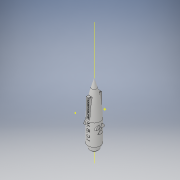
# Autodesk Inventor part: Pencil tooper
Saved by Autodesk Inventor 2018 (Build 220112000, 112)
## iProperties
Created: 2019-05-21
Part Number: Pencil tooper
Material: Generic
Document SubType Name: Modeling
Designer: 10043883
Density: 1 g/cm^3
Appearance: Default
Author: 10043883
Autodesk Inventor part; units mm, degrees
ref_plane "YZ Plane" through (0, 0, 0) normal (1, 0, 0) x (0, 1, 0)
sketch "Sketch1" plane through (0, 0, 0) normal (0, 0, 1) x (1, 0, 0)
  line L0 (0, 36.6275) -> (57.853, 36.6275) construction
  line L1 (25.9989, -2.9024) -> (51.3989, -2.9024)
  line L2 (25.9989, -2.9024) -> (51.3989, -2.9024)
  line L3 (51.3989, -2.9024) -> (51.3989, 38.3311)
  line L4 (51.3989, 38.3311) -> (25.9989, 38.3311)
  line L5 (25.9989, 38.3311) -> (25.9989, -2.9024)
  line L6 (38.6989, -2.9024) -> (38.6989, 38.3311)
  line L7 (25.9989, 38.3311) -> (38.6989, 82.474)
  line L8 (38.6989, 82.474) -> (51.3989, 38.3311)
  line L9 (38.6989, 82.474) -> (38.6989, 38.3311)
  line L10 (51.3989, -2.9024) -> (25.9989, -2.9024)
  line L11 (25.9989, -2.9024) -> (25.9989, -44.3081)
  line L12 (25.9989, -44.3081) -> (51.3989, -44.3081)
  line L13 (51.3989, -44.3081) -> (51.3989, -2.9024)
  line L14 (38.6989, -2.9024) -> (38.6989, -44.3081)
  point P0 (0, 0)
  point P1 (60.1022, 36.6275)
  point P2 (86.4535, -44.3081)
  dimension "d42" = 25.4
  constraints: 30 end point, 4 horizontal, 4 midpoint, 4 parallel, 3 point on line, 2 perpendicular, 1 collinear
  measures "d42" distance of L11.end L12.end
sketch "Sketch2" plane through (0, 0, 0) normal (0, 0, 1) x (1, 0, 0)
  point P0 (0, 0)
revolve "Revolution2" add sketch "Sketch1" angle 360 about axis through (38.6989, -2.9024, 0) along (0, 1, 0) contours L5 L4 L6 L1
revolve "Revolution5" add sketch "Sketch1" angle 360 about axis through (38.6989, 82.474, 0) along (0, -1, 0) contours L1 L14 L12 L11 | L7 L9 L4
hole "Hole4" at (38.6989, -44.3081, 0) direction (0, 1, 0) diameter 10.16 depth 38.1 tip angle 60
ref_plane "Work Plane9" through (38.6989, 17.7144, 12.7) normal (0, 0, -1) x (-1, 0, 0)
ref_plane "Work Plane8" through (38.6989, -44.3081, 0) normal (0, 0, -1) x (0, 1, 0)
sketch "Sketch6" plane through (38.6989, 17.7144, 12.7) normal (0, 0, -1) x (-1, 0, 0)
  line L0 (-3.4954, -41.6942) -> (-3.4954, -36.5195) construction
  line L1 (-3.4954, -36.5195) -> (31.8486, -36.5195) construction
  line L2 (31.8486, -36.5195) -> (31.8486, -41.6942) construction
  line L3 (31.8486, -41.6942) -> (-3.4954, -41.6942) construction
  line L4 (2.6638, -40.6345) -> (-3.4322, -40.6345)
  line L5 (-3.4322, -40.6345) -> (-3.4322, -40.3039)
  line L6 (-3.4322, -40.3039) -> (2.6638, -40.3039)
  line L7 (2.6638, -40.3039) -> (2.6638, -40.6345)
  line L8 (2.7805, -37.7275) -> (2.2846, -38.2525)
  line L9 (2.2846, -38.2525) -> (1.7791, -37.7275)
  line L10 (1.7791, -37.7275) -> (2.2846, -37.2073)
  line L11 (2.2846, -37.2073) -> (2.7805, -37.7275)
  line L12 (1.152, -30.7467) -> (1.8228, -31.087)
  line L13 (1.8228, -31.087) -> (2.4208, -31.7044)
  line L14 (2.4208, -31.7044) -> (2.7173, -32.3461)
  line L15 (2.7173, -32.3461) -> (2.7173, -33.5857)
  line L16 (2.7173, -33.5857) -> (2.4208, -34.2225)
  line L17 (2.4208, -34.2225) -> (1.8228, -34.8447)
  line L18 (1.8228, -34.8447) -> (1.22, -35.1413)
  line L19 (1.22, -35.1413) -> (0.345, -35.4475)
  line L20 (0.345, -35.4475) -> (-1.1085, -35.4475)
  line L21 (-1.1085, -35.4475) -> (-1.9884, -35.1413)
  line L22 (-1.9884, -35.1413) -> (-2.5912, -34.8447)
  line L23 (-2.5912, -34.8447) -> (-3.1891, -34.2225)
  line L24 (-3.1891, -34.2225) -> (-3.4954, -33.5857)
  line L25 (-3.4954, -33.5857) -> (-3.4954, -32.3461)
  line L26 (-3.4954, -32.3461) -> (-3.1891, -31.7044)
  line L27 (-3.1891, -31.7044) -> (-2.5912, -31.087)
  line L28 (-2.5912, -31.087) -> (-1.9203, -30.7467)
  line L29 (-1.9203, -30.7467) -> (-1.7599, -31.0384)
  line L30 (-1.7599, -31.0384) -> (-2.3919, -31.369)
  line L31 (-2.3919, -31.369) -> (-2.9169, -31.9086)
  line L32 (-2.9169, -31.9086) -> (-3.1697, -32.4238)
  line L33 (-3.1697, -32.4238) -> (-3.1697, -33.503)
  line L34 (-3.1697, -33.503) -> (-2.9169, -34.0232)
  line L35 (-2.9169, -34.0232) -> (-2.3919, -34.5628)
  line L36 (-2.3919, -34.5628) -> (-1.8669, -34.8399)
  line L37 (-1.8669, -34.8399) -> (-1.0647, -35.1121)
  line L38 (-1.0647, -35.1121) -> (0.2964, -35.1121)
  line L39 (0.2964, -35.1121) -> (1.0985, -34.8399)
  line L40 (1.0985, -34.8399) -> (1.6235, -34.5628)
  line L41 (1.6235, -34.5628) -> (2.1485, -34.0232)
  line L42 (2.1485, -34.0232) -> (2.4013, -33.503)
  line L43 (2.4013, -33.503) -> (2.4013, -32.4238)
  line L44 (2.4013, -32.4238) -> (2.1485, -31.9086)
  line L45 (2.1485, -31.9086) -> (1.6235, -31.369)
  line L46 (1.6235, -31.369) -> (0.9916, -31.0384)
  line L47 (0.9916, -31.0384) -> (1.152, -30.7467)
  line L48 (2.7805, -27.3244) -> (2.2846, -27.8494)
  line L49 (2.2846, -27.8494) -> (1.7791, -27.3244)
  line L50 (1.7791, -27.3244) -> (2.2846, -26.8042)
  line L51 (2.2846, -26.8042) -> (2.7805, -27.3244)
  line L52 (-0.5251, -21.4569) -> (-0.389, -21.0291)
  line L53 (-0.389, -21.0291) -> (-0.0585, -20.6839)
  line L54 (-0.0585, -20.6839) -> (0.5638, -20.368)
  line L55 (0.5638, -20.368) -> (1.4825, -20.368)
  line L56 (1.4825, -20.368) -> (2.0999, -20.6839)
  line L57 (2.0999, -20.6839) -> (2.4256, -21.0291)
  line L58 (2.4256, -21.0291) -> (2.7173, -21.9576)
  line L59 (2.7173, -21.9576) -> (2.7173, -24.7528)
  line L60 (2.7173, -24.7528) -> (-3.4954, -24.7528)
  line L61 (-3.4954, -24.7528) -> (-3.4954, -21.9576)
  line L62 (-3.4954, -21.9576) -> (-3.194, -21.0291)
  line L63 (-3.194, -21.0291) -> (-2.8731, -20.6839)
  line L64 (-2.8731, -20.6839) -> (-2.246, -20.368)
  line L65 (-2.246, -20.368) -> (-1.6092, -20.368)
  line L66 (-1.6092, -20.368) -> (-0.987, -20.6839)
  line L67 (-0.987, -20.6839) -> (-0.6613, -21.0291)
  line L68 (-0.6613, -21.0291) -> (-0.5251, -21.4569)
  line L69 (-0.3599, -22.0062) -> (-0.3599, -24.4222)
  line L70 (-0.3599, -24.4222) -> (2.4013, -24.4222)
  line L71 (2.4013, -24.4222) -> (2.4013, -22.0062)
  line L72 (2.4013, -22.0062) -> (2.1437, -21.2041)
  line L73 (2.1437, -21.2041) -> (1.9055, -20.9659)
  line L74 (1.9055, -20.9659) -> (1.3999, -20.7034)
  line L75 (1.3999, -20.7034) -> (0.6367, -20.7034)
  line L76 (0.6367, -20.7034) -> (0.136, -20.9659)
  line L77 (0.136, -20.9659) -> (-0.1022, -21.2041)
  line L78 (-0.1022, -21.2041) -> (-0.3599, -22.0062)
  line L79 (-0.6856, -24.4222) -> (-0.6856, -22.0062)
  line L80 (-0.6856, -22.0062) -> (-0.9432, -21.2041)
  line L81 (-0.9432, -21.2041) -> (-1.1863, -20.9659)
  line L82 (-1.1863, -20.9659) -> (-1.687, -20.7034)
  line L83 (-1.687, -20.7034) -> (-2.1683, -20.7034)
  line L84 (-2.1683, -20.7034) -> (-2.6738, -20.9659)
  line L85 (-2.6738, -20.9659) -> (-2.912, -21.2041)
  line L86 (-2.912, -21.2041) -> (-3.1697, -22.0062)
  line L87 (-3.1697, -22.0062) -> (-3.1697, -24.4222)
  line L88 (-3.1697, -24.4222) -> (-0.6856, -24.4222)
  line L89 (2.7805, -16.9213) -> (2.2846, -17.4463)
  line L90 (2.2846, -17.4463) -> (1.7791, -16.9213)
  line L91 (1.7791, -16.9213) -> (2.2846, -16.4012)
  line L92 (2.2846, -16.4012) -> (2.7805, -16.9213)
  line L93 (2.6638, -9.3864) -> (2.6638, -9.717)
  line L94 (2.6638, -9.717) -> (-2.4551, -9.717)
  line L95 (-2.4551, -9.717) -> (2.6638, -11.7295)
  line L96 (2.6638, -11.7295) -> (2.6638, -12.0018)
  line L97 (2.6638, -12.0018) -> (-2.4551, -14.0192)
  line L98 (-2.4551, -14.0192) -> (2.6638, -14.0192)
  line L99 (2.6638, -14.0192) -> (2.6638, -14.3497)
  line L100 (2.6638, -14.3497) -> (-3.4322, -14.3497)
  line L101 (-3.4322, -14.3497) -> (-3.4322, -14.0483)
  line L102 (-3.4322, -14.0483) -> (2.1145, -11.8656)
  line L103 (2.1145, -11.8656) -> (-3.4322, -9.6878)
  line L104 (-3.4322, -9.6878) -> (-3.4322, -9.3864)
  line L105 (-3.4322, -9.3864) -> (2.6638, -9.3864)
  point P0 (38.6989, -17.7144)
  constraints: 2 other
extrude "Extrusion3" add sketch "Sketch6" along normal blind 25.4
ref_plane "Work Plane10" through (51.3989, -2.9024, 0) normal (1, 0, 0) x (0, 1, 0)
fillet "Fillet5" radius 196.85 1 edges at (51.3989, 38.3311, 0)
sketch "Sketch7" plane through (51.3989, -2.9024, 0) normal (1, 0, 0) x (0, 1, 0)
  line L0 (0.2488, 2.5647) -> (0.2488, -2.5647) projected
  circle A0 centre (0.2488, 0) radius 10.3788
  arc A1 (8.5027, 1.9887) -> (1.1594, 9.0888) centre (-0.0471, 0.4934) ccw
  line L1 (1.1594, 9.0888) -> (0.276, 3.4875)
  line L2 (8.5027, 1.9887) -> (2.844, 1.4137)
  arc A2 (2.844, 1.4137) -> (0.276, 3.4875) centre (-0.4963, -0.0957) ccw
  circle A3 centre (0.2488, 0) radius 2.2322
  arc A4 (0.8722, -9.1023) -> (8.4313, -2.2325) centre (-0.0683, -0.4738) ccw
  line L3 (8.4313, -2.2325) -> (2.8987, -0.9894)
  line L4 (0.8722, -9.1023) -> (0.6635, -3.4182)
  arc A5 (0.6635, -3.4182) -> (2.8987, -0.9894) centre (-0.6272, 0.0125) ccw
  arc A6 (-7.9804, 4.8535) -> (-7.5597, -4.9877) centre (-0.6296, 0.2381) ccw
  line L5 (-7.5597, -4.9877) -> (-2.9749, -1.6509)
  line L6 (-7.9804, 4.8535) -> (-2.9749, 1.4137)
  arc A7 (-2.9749, 1.4137) -> (-2.9749, -1.6509) centre (0.355, -0.1186) ccw
  point P0 (2.9024, 0)
  constraints: 12 end point, 12 point on circle, 8 centre point, 1 coincident, 1 midpoint
extrude "Extrusion4" add sketch "Sketch7" against normal blind 25.4 contours A3 L0 | L0 A3 | L2 A2 L1 A1 | L4 A5 L3 A4 | L6 A7 L5 A6
chamfer "Chamfer1" distance 5.715 angle 45 1 edges at (51.3989, -44.3081, 0)
chamfer "Chamfer2" distance 5.715 angle 45 1 edges at (51.3989, -38.5931, 0)
sketch "Sketch8" plane through (38.6989, 17.7144, 12.7) normal (0, 0, -1) x (-1, 0, 0)
  line L0 (-3.3915, 35.5657) -> (3.9696, 35.5657)
  line L1 (3.9696, 35.5657) -> (3.9696, -3.0269)
  line L2 (3.9696, -3.0269) -> (-3.3915, -3.0269)
  line L3 (-3.3915, -3.0269) -> (-3.3915, 35.5657)
  point P0 (38.6989, -17.7144)
  constraints: 8 end point, 2 parallel, 1 horizontal, 1 perpendicular
extrude "Extrusion5" add sketch "Sketch8" along normal blind 25.4
sketch "Sketch9" plane through (38.6989, 17.7144, 12.7) normal (0, 0, 1) x (1, 0, 0)
  line L0 (2.0658, 35.4953) -> (2.0658, 4.9175) construction
  line L1 (2.0658, 4.9175) -> (-2.3913, 4.9175) construction
  line L2 (-2.3913, 4.9175) -> (-2.3913, 35.4953) construction
  line L3 (-2.3913, 35.4953) -> (2.0658, 35.4953) construction
  line L4 (1.4194, 33.6183) -> (-0.8902, 33.6183)
  spline S0 degree 2 poles (-0.8902, 33.6183) (-0.9598, 33.6183) (-1.0319, 33.5562) (-1.0543, 33.4741) knots 0 0 0 1 2 2 2
  line L5 (-1.0543, 33.4741) -> (-1.1264, 33.4741)
  line L6 (-1.1264, 33.4741) -> (-1.1264, 34.4288)
  line L7 (-1.1264, 34.4288) -> (-1.0543, 34.4288)
  spline S1 degree 2 poles (-1.0543, 34.4288) (-1.0319, 34.3468) (-0.9598, 34.2846) (-0.8902, 34.2846) knots 0 0 0 1 2 2 2
  line L8 (-0.8902, 34.2846) -> (1.4194, 34.2846)
  line L9 (1.4194, 34.2846) -> (1.4194, 35.2293)
  spline S2 degree 2 poles (1.4194, 35.2293) (1.4194, 35.2965) (1.3573, 35.3686) (1.2752, 35.3909) knots 0 0 0 1 2 2 2
  line L10 (1.2752, 35.3909) -> (1.2752, 35.463)
  line L11 (1.2752, 35.463) -> (2.0658, 35.463)
  line L12 (2.0658, 35.463) -> (2.0658, 35.3909)
  spline S3 degree 2 poles (2.0658, 35.3909) (1.9838, 35.3661) (1.9216, 35.2965) (1.9216, 35.2293) knots 0 0 0 1 2 2 2
  line L13 (1.9216, 35.2293) -> (1.9216, 32.6761)
  spline S4 degree 2 poles (1.9216, 32.6761) (1.9216, 32.6065) (1.9838, 32.5344) (2.0658, 32.512) knots 0 0 0 1 2 2 2
  line L14 (2.0658, 32.512) -> (2.0658, 32.4399)
  line L15 (2.0658, 32.4399) -> (1.2752, 32.4399)
  line L16 (1.2752, 32.4399) -> (1.2752, 32.512)
  spline S5 degree 2 poles (1.2752, 32.512) (1.3573, 32.5344) (1.4194, 32.6065) (1.4194, 32.6736) knots 0 0 0 1 2 2 2
  line L17 (1.4194, 32.6736) -> (1.4194, 33.6183)
  line L18 (-0.4999, 30.2968) -> (-0.4999, 31.4429)
  line L19 (-0.4999, 31.4429) -> (-0.7733, 31.5722)
  spline S6 degree 2 poles (-0.7733, 31.5722) (-0.8728, 31.6195) (-0.9275, 31.6195) knots 0 0 0 1 1 1
  spline S7 degree 2 poles (-0.9275, 31.6195) (-1.0344, 31.6195) (-1.0642, 31.4753) knots 0 0 0 1 1 1
  line L20 (-1.0642, 31.4753) -> (-1.1264, 31.4753)
  line L21 (-1.1264, 31.4753) -> (-1.1264, 32.3976)
  line L22 (-1.1264, 32.3976) -> (-1.0642, 32.3976)
  spline S8 degree 2 poles (-1.0642, 32.3976) (-1.0518, 32.3131) (-0.9747, 32.2311) (-0.8628, 32.1739) knots 0 0 0 1 2 2 2
  line L23 (-0.8628, 32.1739) -> (0.9869, 31.2615)
  spline S9 degree 2 poles (0.9869, 31.2615) (1.0913, 31.2093) (1.1708, 31.2093) knots 0 0 0 1 1 1
  spline S10 degree 2 poles (1.1708, 31.2093) (1.2603, 31.2093) (1.3125, 31.3336) knots 0 0 0 1 1 1
  line L24 (1.3125, 31.3336) -> (1.3747, 31.3336)
  line L25 (1.3747, 31.3336) -> (1.3747, 30.364)
  line L26 (1.3747, 30.364) -> (1.3125, 30.364)
  spline S11 degree 2 poles (1.3125, 30.364) (1.2628, 30.4858) (1.1609, 30.4858) knots 0 0 0 1 1 1
  spline S12 degree 2 poles (1.1609, 30.4858) (1.0863, 30.4858) (0.9794, 30.4311) knots 0 0 0 1 1 1
  line L27 (0.9794, 30.4311) -> (-0.8131, 29.4839)
  spline S13 degree 2 poles (-0.8131, 29.4839) (-0.9598, 29.4068) (-1.0468, 29.3173) (-1.0642, 29.2253) knots 0 0 0 1 2 2 2
  line L28 (-1.0642, 29.2253) -> (-1.1264, 29.2253)
  line L29 (-1.1264, 29.2253) -> (-1.1264, 30.2471)
  line L30 (-1.1264, 30.2471) -> (-1.0642, 30.2471)
  spline S14 degree 2 poles (-1.0642, 30.2471) (-1.0393, 30.1029) (-0.9275, 30.1029) knots 0 0 0 1 1 1
  spline S15 degree 2 poles (-0.9275, 30.1029) (-0.8579, 30.1029) (-0.7559, 30.1576) knots 0 0 0 1 1 1
  line L31 (-0.7559, 30.1576) -> (-0.4999, 30.2968)
  line L32 (-0.1493, 30.4758) -> (0.6512, 30.8836)
  line L33 (0.6512, 30.8836) -> (-0.1493, 31.2714)
  line L34 (-0.1493, 31.2714) -> (-0.1493, 30.4758)
  line L35 (-0.0971, 28.2731) -> (-0.8976, 28.2731)
  spline S16 degree 2 poles (-0.8976, 28.2731) (-0.9648, 28.2731) (-1.0393, 28.211) (-1.0642, 28.1289) knots 0 0 0 1 2 2 2
  line L36 (-1.0642, 28.1289) -> (-1.1264, 28.1289)
  line L37 (-1.1264, 28.1289) -> (-1.1264, 29.0165)
  line L38 (-1.1264, 29.0165) -> (-1.0642, 29.0165)
  spline S17 degree 2 poles (-1.0642, 29.0165) (-1.0443, 28.9369) (-0.9672, 28.8723) (-0.9001, 28.8723) knots 0 0 0 1 2 2 2
  line L39 (-0.9001, 28.8723) -> (1.1485, 28.8723)
  spline S18 degree 2 poles (1.1485, 28.8723) (1.2156, 28.8723) (1.2877, 28.9344) (1.3125, 29.0165) knots 0 0 0 1 2 2 2
  line L40 (1.3125, 29.0165) -> (1.3747, 29.0165)
  line L41 (1.3747, 29.0165) -> (1.3747, 27.3781)
  spline S19 degree 2 poles (1.3747, 27.3781) (1.3747, 27.0574) (1.3101, 26.7243) (1.2255, 26.5925) knots 0 0 0 1 2 2 2
  spline S20 degree 2 poles (1.2255, 26.5925) (1.049, 26.3215) (0.6512, 26.3215) knots 0 0 0 1 1 1
  spline S21 degree 2 poles (0.6512, 26.3215) (0.3479, 26.3215) (0.0048, 26.6547) (-0.0698, 27.0251) knots 0 0 0 1 2 2 2
  line L42 (-0.0698, 27.0251) -> (-0.7311, 26.5527)
  spline S22 degree 2 poles (-0.7311, 26.5527) (-0.915, 26.421) (-1.0468, 26.2668) (-1.0642, 26.1699) knots 0 0 0 1 2 2 2
  line L43 (-1.0642, 26.1699) -> (-1.1264, 26.1699)
  line L44 (-1.1264, 26.1699) -> (-1.1264, 27.219)
  line L45 (-1.1264, 27.219) -> (-1.0642, 27.219)
  spline S23 degree 2 poles (-1.0642, 27.219) (-1.0319, 27.1046) (-0.9648, 27.1046) knots 0 0 0 1 1 1
  spline S24 degree 2 poles (-0.9648, 27.1046) (-0.915, 27.1046) (-0.8131, 27.1767) knots 0 0 0 1 1 1
  line L46 (-0.8131, 27.1767) -> (-0.0971, 27.674)
  line L47 (-0.0971, 27.674) -> (-0.0971, 28.2731)
  line L48 (0.3554, 28.2731) -> (0.3554, 27.3731)
  spline S25 degree 2 poles (0.3554, 27.3731) (0.3554, 27.1668) (0.4001, 27.0698) knots 0 0 0 1 1 1
  spline S26 degree 2 poles (0.4001, 27.0698) (0.4598, 26.9306) (0.6388, 26.9306) knots 0 0 0 1 1 1
  spline S27 degree 2 poles (0.6388, 26.9306) (0.7979, 26.9306) (0.9222, 27.1245) (0.9222, 27.3731) knots 0 0 0 1 2 2 2
  line L49 (0.9222, 27.3731) -> (0.9222, 28.2731)
  line L50 (0.9222, 28.2731) -> (0.3554, 28.2731)
  line L51 (-0.1617, 23.6216) -> (-0.1617, 24.1909)
  spline S28 degree 2 poles (-0.1617, 24.1909) (-0.1617, 24.263) (-0.2239, 24.3376) (-0.3059, 24.36) knots 0 0 0 1 2 2 2
  line L52 (-0.3059, 24.36) -> (-0.3059, 24.4196)
  line L53 (-0.3059, 24.4196) -> (0.3604, 24.4196)
  line L54 (0.3604, 24.4196) -> (0.3604, 24.36)
  spline S29 degree 2 poles (0.3604, 24.36) (0.2808, 24.3376) (0.2162, 24.263) (0.2162, 24.1934) knots 0 0 0 1 2 2 2
  line L55 (0.2162, 24.1934) -> (0.2162, 23)
  line L56 (0.2162, 23) -> (0.1515, 23)
  spline S30 degree 2 poles (0.1515, 23) (0.1291, 23.0796) (0.0446, 23.1442) (-0.0349, 23.1442) knots 0 0 0 1 2 2 2
  line L57 (-0.0349, 23.1442) -> (-0.562, 23.1442)
  spline S31 degree 2 poles (-0.562, 23.1442) (-0.6291, 23.1442) (-0.7062, 23.0796) (-0.7286, 23) knots 0 0 0 1 2 2 2
  line L58 (-0.7286, 23) -> (-0.7808, 23)
  spline S32 degree 2 poles (-0.7808, 23) (-1.1811, 23.7235) (-1.1811, 24.442) knots 0 0 0 1 1 1
  spline S33 degree 2 poles (-1.1811, 24.442) (-1.1811, 25.0635) (-0.8877, 25.4464) knots 0 0 0 1 1 1
  spline S34 degree 2 poles (-0.8877, 25.4464) (-0.7286, 25.6552) (-0.4899, 25.782) knots 0 0 0 1 1 1
  spline S35 degree 2 poles (-0.4899, 25.782) (-0.209, 25.9312) (0.1117, 25.9312) knots 0 0 0 1 1 1
  spline S36 degree 2 poles (0.1117, 25.9312) (0.5543, 25.9312) (0.8974, 25.6602) knots 0 0 0 1 1 1
  spline S37 degree 2 poles (0.8974, 25.6602) (1.4294, 25.2351) (1.4294, 24.4072) knots 0 0 0 1 1 1
  spline S38 degree 2 poles (1.4294, 24.4072) (1.4294, 24.0417) (1.2678, 23.5768) knots 0 0 0 1 1 1
  spline S39 degree 2 poles (1.2678, 23.5768) (1.2056, 23.3904) (1.2056, 23.3605) knots 0 0 0 1 1 1
  spline S40 degree 2 poles (1.2056, 23.3605) (1.2056, 23.3232) (1.2429, 23.271) knots 0 0 0 1 1 1
  line L59 (1.2429, 23.271) -> (1.2131, 23.2163)
  line L60 (1.2131, 23.2163) -> (0.5841, 23.5122)
  line L61 (0.5841, 23.5122) -> (0.609, 23.5669)
  spline S41 degree 2 poles (0.609, 23.5669) (0.6189, 23.5669) (0.6239, 23.5669) knots 0 0 0 1 1 1
  spline S42 degree 2 poles (0.6239, 23.5669) (0.7059, 23.5669) (0.7929, 23.731) knots 0 0 0 1 1 1
  spline S43 degree 2 poles (0.7929, 23.731) (0.957, 24.0368) (0.957, 24.3873) knots 0 0 0 1 1 1
  spline S44 degree 2 poles (0.957, 24.3873) (0.957, 24.7901) (0.7358, 25.0511) knots 0 0 0 1 1 1
  spline S45 degree 2 poles (0.7358, 25.0511) (0.5021, 25.3221) (0.1093, 25.3221) knots 0 0 0 1 1 1
  spline S46 degree 2 poles (0.1093, 25.3221) (-0.2612, 25.3221) (-0.4824, 25.0735) knots 0 0 0 1 1 1
  spline S47 degree 2 poles (-0.4824, 25.0735) (-0.7087, 24.8199) (-0.7087, 24.36) knots 0 0 0 1 1 1
  spline S48 degree 2 poles (-0.7087, 24.36) (-0.7087, 23.9224) (-0.5446, 23.6216) knots 0 0 0 1 1 1
  line L62 (-0.5446, 23.6216) -> (-0.1617, 23.6216)
  line L63 (-0.0623, 21.839) -> (-0.6739, 21.839)
  line L64 (-0.6739, 21.839) -> (-0.6739, 20.2504)
  spline S49 degree 2 poles (-0.6739, 20.2504) (-0.6739, 20.1832) (-0.6117, 20.1087) (-0.5297, 20.0863) knots 0 0 0 1 2 2 2
  line L65 (-0.5297, 20.0863) -> (-0.5297, 20.0241)
  line L66 (-0.5297, 20.0241) -> (-1.2706, 20.0241)
  line L67 (-1.2706, 20.0241) -> (-1.2706, 20.0863)
  spline S50 degree 2 poles (-1.2706, 20.0863) (-1.191, 20.1062) (-1.1264, 20.1832) (-1.1264, 20.2529) knots 0 0 0 1 2 2 2
  line L68 (-1.1264, 20.2529) -> (-1.1264, 22.5824)
  line L69 (-1.1264, 22.5824) -> (-1.0642, 22.5824)
  spline S51 degree 2 poles (-1.0642, 22.5824) (-1.0443, 22.5028) (-0.9672, 22.4382) (-0.9001, 22.4382) knots 0 0 0 1 2 2 2
  line L70 (-0.9001, 22.4382) -> (1.1485, 22.4382)
  spline S52 degree 2 poles (1.1485, 22.4382) (1.2156, 22.4382) (1.2877, 22.5003) (1.3125, 22.5824) knots 0 0 0 1 2 2 2
  line L71 (1.3125, 22.5824) -> (1.3747, 22.5824)
  line L72 (1.3747, 22.5824) -> (1.3747, 20.32)
  spline S53 degree 2 poles (1.3747, 20.32) (1.3747, 20.2504) (1.4368, 20.1758) (1.5189, 20.1534) knots 0 0 0 1 2 2 2
  line L73 (1.5189, 20.1534) -> (1.5189, 20.0937)
  line L74 (1.5189, 20.0937) -> (0.778, 20.0937)
  line L75 (0.778, 20.0937) -> (0.778, 20.1534)
  spline S54 degree 2 poles (0.778, 20.1534) (0.8601, 20.1758) (0.9222, 20.2504) (0.9222, 20.32) knots 0 0 0 1 2 2 2
  line L76 (0.9222, 20.32) -> (0.9222, 21.839)
  line L77 (0.9222, 21.839) -> (0.3728, 21.839)
  line L78 (0.3728, 21.839) -> (0.3728, 20.8943)
  spline S55 degree 2 poles (0.3728, 20.8943) (0.3728, 20.8272) (0.4349, 20.7526) (0.517, 20.7277) knots 0 0 0 1 2 2 2
  line L79 (0.517, 20.7277) -> (0.517, 20.668)
  line L80 (0.517, 20.668) -> (-0.2065, 20.668)
  line L81 (-0.2065, 20.668) -> (-0.2065, 20.7277)
  spline S56 degree 2 poles (-0.2065, 20.7277) (-0.1269, 20.7501) (-0.0623, 20.8247) (-0.0623, 20.8943) knots 0 0 0 1 2 2 2
  line L82 (-0.0623, 20.8943) -> (-0.0623, 21.839)
  line L83 (0.9222, 18.2664) -> (-0.8976, 18.2664)
  spline S57 degree 2 poles (-0.8976, 18.2664) (-0.9648, 18.2664) (-1.0393, 18.2043) (-1.0642, 18.1222) knots 0 0 0 1 2 2 2
  line L84 (-1.0642, 18.1222) -> (-1.1264, 18.1222)
  line L85 (-1.1264, 18.1222) -> (-1.1264, 19.0098)
  line L86 (-1.1264, 19.0098) -> (-1.0642, 19.0098)
  spline S58 degree 2 poles (-1.0642, 19.0098) (-1.0443, 18.9302) (-0.9672, 18.8656) (-0.8976, 18.8656) knots 0 0 0 1 2 2 2
  line L87 (-0.8976, 18.8656) -> (0.9222, 18.8656)
  line L88 (0.9222, 18.8656) -> (0.9222, 19.604)
  spline S59 degree 2 poles (0.9222, 19.604) (0.9222, 19.6736) (0.8576, 19.7482) (0.778, 19.7705) knots 0 0 0 1 2 2 2
  line L89 (0.778, 19.7705) -> (0.778, 19.8302)
  line L90 (0.778, 19.8302) -> (1.5189, 19.8302)
  line L91 (1.5189, 19.8302) -> (1.5189, 19.7705)
  spline S60 degree 2 poles (1.5189, 19.7705) (1.4393, 19.7507) (1.3747, 19.6761) (1.3747, 19.604) knots 0 0 0 1 2 2 2
  line L92 (1.3747, 19.604) -> (1.3747, 17.5281)
  spline S61 degree 2 poles (1.3747, 17.5281) (1.3747, 17.4584) (1.4368, 17.3839) (1.5189, 17.3615) knots 0 0 0 1 2 2 2
  line L93 (1.5189, 17.3615) -> (1.5189, 17.3018)
  line L94 (1.5189, 17.3018) -> (0.778, 17.3018)
  line L95 (0.778, 17.3018) -> (0.778, 17.3615)
  spline S62 degree 2 poles (0.778, 17.3615) (0.8576, 17.3839) (0.9222, 17.4584) (0.9222, 17.5281) knots 0 0 0 1 2 2 2
  line L96 (0.9222, 17.5281) -> (0.9222, 18.2664)
  spline S63 degree 2 poles (1.4294, 16.5585) (1.4294, 16.4043) (1.2156, 16.193) (1.0614, 16.193) knots 0 0 0 1 2 2 2
  spline S64 degree 2 poles (1.0614, 16.193) (0.9098, 16.193) (0.696, 16.4093) (0.696, 16.5585) knots 0 0 0 1 2 2 2
  spline S65 degree 2 poles (0.696, 16.5585) (0.696, 16.7126) (0.9123, 16.9264) (1.0639, 16.9264) knots 0 0 0 1 2 2 2
  spline S66 degree 2 poles (1.0639, 16.9264) (1.2156, 16.9264) (1.4269, 16.7151) (1.4294, 16.5585) knots 0 0 0 1 2 2 2
  spline S67 degree 2 poles (-0.4476, 16.5585) (-0.4476, 16.4043) (-0.6615, 16.193) (-0.8156, 16.193) knots 0 0 0 1 2 2 2
  spline S68 degree 2 poles (-0.8156, 16.193) (-0.9672, 16.193) (-1.1811, 16.4093) (-1.1811, 16.5585) knots 0 0 0 1 2 2 2
  spline S69 degree 2 poles (-1.1811, 16.5585) (-1.1811, 16.7126) (-0.9648, 16.9264) (-0.8131, 16.9264) knots 0 0 0 1 2 2 2
  spline S70 degree 2 poles (-0.8131, 16.9264) (-0.6615, 16.9264) (-0.4501, 16.7151) (-0.4476, 16.5585) knots 0 0 0 1 2 2 2
  line L97 (-1.1264, 13.7069) -> (0.9794, 14.8331)
  line L98 (0.9794, 14.8331) -> (-0.8902, 14.8331)
  spline S71 degree 2 poles (-0.8902, 14.8331) (-0.9598, 14.8331) (-1.0319, 14.7709) (-1.0543, 14.6889) knots 0 0 0 1 2 2 2
  line L99 (-1.0543, 14.6889) -> (-1.1264, 14.6889)
  line L100 (-1.1264, 14.6889) -> (-1.1264, 15.5864)
  line L101 (-1.1264, 15.5864) -> (-1.0543, 15.5864)
  spline S72 degree 2 poles (-1.0543, 15.5864) (-1.0319, 15.5043) (-0.9598, 15.4422) (-0.8902, 15.4422) knots 0 0 0 1 2 2 2
  line L102 (-0.8902, 15.4422) -> (1.6879, 15.4422)
  spline S73 degree 2 poles (1.6879, 15.4422) (1.7551, 15.4422) (1.8272, 15.5043) (1.8495, 15.5864) knots 0 0 0 1 2 2 2
  line L103 (1.8495, 15.5864) -> (1.9216, 15.5864)
  line L104 (1.9216, 15.5864) -> (1.9216, 14.4104)
  line L105 (1.9216, 14.4104) -> (1.8495, 14.4104)
  spline S74 degree 2 poles (1.8495, 14.4104) (1.8222, 14.5149) (1.7277, 14.5149) knots 0 0 0 1 1 1
  spline S75 degree 2 poles (1.7277, 14.5149) (1.683, 14.5149) (1.6233, 14.485) knots 0 0 0 1 1 1
  line L106 (1.6233, 14.485) -> (0.0546, 13.6547)
  line L107 (0.0546, 13.6547) -> (1.5984, 12.8119)
  spline S76 degree 2 poles (1.5984, 12.8119) (1.7004, 12.7547) (1.7476, 12.7547) knots 0 0 0 1 1 1
  spline S77 degree 2 poles (1.7476, 12.7547) (1.8396, 12.7547) (1.8495, 12.8666) knots 0 0 0 1 1 1
  line L108 (1.8495, 12.8666) -> (1.9216, 12.8666)
  line L109 (1.9216, 12.8666) -> (1.9216, 11.713)
  line L110 (1.9216, 11.713) -> (1.8495, 11.713)
  spline S78 degree 2 poles (1.8495, 11.713) (1.8272, 11.795) (1.7551, 11.8572) (1.6879, 11.8572) knots 0 0 0 1 2 2 2
  line L111 (1.6879, 11.8572) -> (-0.8902, 11.8572)
  spline S79 degree 2 poles (-0.8902, 11.8572) (-0.9598, 11.8572) (-1.0319, 11.795) (-1.0543, 11.713) knots 0 0 0 1 2 2 2
  line L112 (-1.0543, 11.713) -> (-1.1264, 11.713)
  line L113 (-1.1264, 11.713) -> (-1.1264, 12.6677)
  line L114 (-1.1264, 12.6677) -> (-1.0543, 12.6677)
  spline S80 degree 2 poles (-1.0543, 12.6677) (-1.0344, 12.5881) (-0.9598, 12.5235) (-0.8902, 12.5235) knots 0 0 0 1 2 2 2
  line L115 (-0.8902, 12.5235) -> (0.9794, 12.5235)
  line L116 (0.9794, 12.5235) -> (-1.1264, 13.7069)
  line L117 (1.6656, 8.3269) -> (0.9471, 8.6899)
  line L118 (0.9471, 8.6899) -> (0.9844, 8.752)
  spline S81 degree 2 poles (0.9844, 8.752) (1.0067, 8.7495) (1.0192, 8.7495) knots 0 0 0 1 1 1
  spline S82 degree 2 poles (1.0192, 8.7495) (1.0962, 8.7495) (1.1833, 8.8788) knots 0 0 0 1 1 1
  spline S83 degree 2 poles (1.1833, 8.8788) (1.4592, 9.2766) (1.4592, 9.8136) knots 0 0 0 1 1 1
  spline S84 degree 2 poles (1.4592, 9.8136) (1.4592, 10.0498) (1.402, 10.2313) knots 0 0 0 1 1 1
  spline S85 degree 2 poles (1.402, 10.2313) (1.3573, 10.363) (1.1783, 10.5271) (1.0714, 10.5271) knots 0 0 0 1 2 2 2
  spline S86 degree 2 poles (1.0714, 10.5271) (0.8998, 10.5271) (0.8377, 10.3183) knots 0 0 0 1 1 1
  spline S87 degree 2 poles (0.8377, 10.3183) (0.8079, 10.2114) (0.7706, 9.8583) knots 0 0 0 1 1 1
  line L119 (0.7706, 9.8583) -> (0.7358, 9.5078)
  spline S88 degree 2 poles (0.7358, 9.5078) (0.701, 9.197) (0.5866, 8.8092) (0.4797, 8.66) knots 0 0 0 1 2 2 2
  spline S89 degree 2 poles (0.4797, 8.66) (0.3703, 8.5084) (0.0148, 8.3318) (-0.1891, 8.3318) knots 0 0 0 1 2 2 2
  spline S90 degree 2 poles (-0.1891, 8.3318) (-0.5098, 8.3318) (-0.7609, 8.5407) knots 0 0 0 1 1 1
  spline S91 degree 2 poles (-0.7609, 8.5407) (-0.9896, 8.7271) (-1.099, 9.1224) knots 0 0 0 1 1 1
  spline S92 degree 2 poles (-1.099, 9.1224) (-1.1811, 9.4183) (-1.1811, 9.7539) knots 0 0 0 1 1 1
  spline S93 degree 2 poles (-1.1811, 9.7539) (-1.1811, 10.3605) (-0.8902, 10.9497) knots 0 0 0 1 1 1
  spline S94 degree 2 poles (-0.8902, 10.9497) (-0.833, 11.0741) (-0.833, 11.0989) knots 0 0 0 1 1 1
  spline S95 degree 2 poles (-0.833, 11.0989) (-0.833, 11.1287) (-0.8827, 11.1909) knots 0 0 0 1 1 1
  line L120 (-0.8827, 11.1909) -> (-0.8479, 11.2555)
  line L121 (-0.8479, 11.2555) -> (-0.1021, 10.9249)
  line L122 (-0.1021, 10.9249) -> (-0.1319, 10.8602)
  spline S96 degree 2 poles (-0.1319, 10.8602) (-0.1518, 10.8602) (-0.1617, 10.8602) knots 0 0 0 1 1 1
  spline S97 degree 2 poles (-0.1617, 10.8602) (-0.2612, 10.8602) (-0.3457, 10.7633) knots 0 0 0 1 1 1
  spline S98 degree 2 poles (-0.3457, 10.7633) (-0.4775, 10.6191) (-0.6639, 10.0125) (-0.6639, 9.739) knots 0 0 0 1 2 2 2
  spline S99 degree 2 poles (-0.6639, 9.739) (-0.6639, 9.4431) (-0.5645, 9.2318) knots 0 0 0 1 1 1
  spline S100 degree 2 poles (-0.5645, 9.2318) (-0.5073, 9.1175) (-0.3209, 8.9782) (-0.2214, 8.9782) knots 0 0 0 1 2 2 2
  spline S101 degree 2 poles (-0.2214, 8.9782) (-0.0698, 8.9782) (-0.0051, 9.1423) knots 0 0 0 1 1 1
  spline S102 degree 2 poles (-0.0051, 9.1423) (0.0396, 9.2542) (0.0794, 9.6023) knots 0 0 0 1 1 1
  line L123 (0.0794, 9.6023) -> (0.1142, 9.9453)
  spline S103 degree 2 poles (0.1142, 9.9453) (0.1515, 10.2909) (0.2162, 10.5768) (0.2858, 10.7185) knots 0 0 0 1 2 2 2
  spline S104 degree 2 poles (0.2858, 10.7185) (0.3877, 10.9224) (0.5891, 11.0392) knots 0 0 0 1 1 1
  spline S105 degree 2 poles (0.5891, 11.0392) (0.7706, 11.1437) (1.0043, 11.1437) knots 0 0 0 1 1 1
  spline S106 degree 2 poles (1.0043, 11.1437) (1.3896, 11.1437) (1.6432, 10.8776) knots 0 0 0 1 1 1
  spline S107 degree 2 poles (1.6432, 10.8776) (1.9763, 10.5296) (1.9763, 9.831) knots 0 0 0 1 1 1
  spline S108 degree 2 poles (1.9763, 9.831) (1.9763, 9.5376) (1.857, 9.0329) (1.6979, 8.6575) knots 0 0 0 1 2 2 2
  spline S109 degree 2 poles (1.6979, 8.6575) (1.6482, 8.5258) (1.6482, 8.4984) knots 0 0 0 1 1 1
  spline S110 degree 2 poles (1.6482, 8.4984) (1.6482, 8.4512) (1.6979, 8.389) knots 0 0 0 1 1 1
  line L124 (1.6979, 8.389) -> (1.6656, 8.3269)
  line L125 (-1.0095, 8.133) -> (-0.2388, 7.8471)
  line L126 (-0.2388, 7.8471) -> (-0.2637, 7.7799)
  spline S111 degree 2 poles (-0.2637, 7.7799) (-0.291, 7.7824) (-0.3084, 7.7824) knots 0 0 0 1 1 1
  spline S112 degree 2 poles (-0.3084, 7.7824) (-0.4004, 7.7824) (-0.4775, 7.668) knots 0 0 0 1 1 1
  spline S113 degree 2 poles (-0.4775, 7.668) (-0.557, 7.5487) (-0.6639, 7.1435) (-0.6639, 6.9595) knots 0 0 0 1 2 2 2
  spline S114 degree 2 poles (-0.6639, 6.9595) (-0.6639, 6.6587) (-0.5272, 6.5244) knots 0 0 0 1 1 1
  spline S115 degree 2 poles (-0.5272, 6.5244) (-0.4576, 6.4548) (-0.2686, 6.4051) (-0.0772, 6.4051) knots 0 0 0 1 2 2 2
  line L127 (-0.0772, 6.4051) -> (1.6855, 6.4051)
  spline S116 degree 2 poles (1.6855, 6.4051) (1.7551, 6.4051) (1.8272, 6.4672) (1.8495, 6.5493) knots 0 0 0 1 2 2 2
  line L128 (1.8495, 6.5493) -> (1.9216, 6.5493)
  line L129 (1.9216, 6.5493) -> (1.9216, 5.5946)
  line L130 (1.9216, 5.5946) -> (1.8495, 5.5946)
  spline S117 degree 2 poles (1.8495, 5.5946) (1.8272, 5.6767) (1.7551, 5.7388) (1.6855, 5.7388) knots 0 0 0 1 2 2 2
  line L131 (1.6855, 5.7388) -> (-0.1095, 5.7388)
  spline S118 degree 2 poles (-0.1095, 5.7388) (-0.5521, 5.7388) (-0.7485, 5.8606) knots 0 0 0 1 1 1
  spline S119 degree 2 poles (-0.7485, 5.8606) (-0.9548, 5.9924) (-1.1811, 6.4996) (-1.1811, 6.8402) knots 0 0 0 1 2 2 2
  spline S120 degree 2 poles (-1.1811, 6.8402) (-1.1811, 7.0341) (-1.1288, 7.32) (-1.0319, 7.6432) knots 0 0 0 1 2 2 2
  spline S121 degree 2 poles (-1.0319, 7.6432) (-0.9747, 7.8446) (-0.9747, 7.9291) knots 0 0 0 1 1 1
  spline S122 degree 2 poles (-0.9747, 7.9291) (-0.9747, 8.0037) (-1.0369, 8.0658) knots 0 0 0 1 1 1
  line L132 (-1.0369, 8.0658) -> (-1.0095, 8.133)
  line L133 (0.2037, 2.5367) -> (0.2037, 4.2944)
  line L134 (0.2037, 4.2944) -> (-0.8927, 4.2944)
  spline S123 degree 2 poles (-0.8927, 4.2944) (-0.9598, 4.2944) (-1.0344, 4.2297) (-1.0543, 4.1502) knots 0 0 0 1 2 2 2
  line L135 (-1.0543, 4.1502) -> (-1.1264, 4.1502)
  line L136 (-1.1264, 4.1502) -> (-1.1264, 5.1048)
  line L137 (-1.1264, 5.1048) -> (-1.0543, 5.1048)
  spline S124 degree 2 poles (-1.0543, 5.1048) (-1.0319, 5.0228) (-0.9598, 4.9607) (-0.8927, 4.9607) knots 0 0 0 1 2 2 2
  line L138 (-0.8927, 4.9607) -> (1.6879, 4.9607)
  spline S125 degree 2 poles (1.6879, 4.9607) (1.7551, 4.9607) (1.8272, 5.0228) (1.8495, 5.1048) knots 0 0 0 1 2 2 2
  line L139 (1.8495, 5.1048) -> (1.9216, 5.1048)
  line L140 (1.9216, 5.1048) -> (1.9216, 4.1502)
  line L141 (1.9216, 4.1502) -> (1.8495, 4.1502)
  spline S126 degree 2 poles (1.8495, 4.1502) (1.8297, 4.2322) (1.7551, 4.2944) (1.6879, 4.2944) knots 0 0 0 1 2 2 2
  line L142 (1.6879, 4.2944) -> (0.7059, 4.2944)
  line L143 (0.7059, 4.2944) -> (0.7059, 2.5367)
  line L144 (0.7059, 2.5367) -> (1.6879, 2.5367)
  spline S127 degree 2 poles (1.6879, 2.5367) (1.7551, 2.5367) (1.8297, 2.5988) (1.8495, 2.6809) knots 0 0 0 1 2 2 2
  line L145 (1.8495, 2.6809) -> (1.9216, 2.6809)
  line L146 (1.9216, 2.6809) -> (1.9216, 1.7262)
  line L147 (1.9216, 1.7262) -> (1.8495, 1.7262)
  spline S128 degree 2 poles (1.8495, 1.7262) (1.8272, 1.8082) (1.7551, 1.8704) (1.6879, 1.8704) knots 0 0 0 1 2 2 2
  line L148 (1.6879, 1.8704) -> (-0.8927, 1.8704)
  spline S129 degree 2 poles (-0.8927, 1.8704) (-0.9598, 1.8704) (-1.0319, 1.8082) (-1.0543, 1.7262) knots 0 0 0 1 2 2 2
  line L149 (-1.0543, 1.7262) -> (-1.1264, 1.7262)
  line L150 (-1.1264, 1.7262) -> (-1.1264, 2.6809)
  line L151 (-1.1264, 2.6809) -> (-1.0543, 2.6809)
  spline S130 degree 2 poles (-1.0543, 2.6809) (-1.0344, 2.6013) (-0.9598, 2.5367) (-0.8927, 2.5367) knots 0 0 0 1 2 2 2
  line L152 (-0.8927, 2.5367) -> (0.2037, 2.5367)
  line L153 (1.6656, -1.6599) -> (0.9471, -1.2969)
  line L154 (0.9471, -1.2969) -> (0.9844, -1.2348)
  spline S131 degree 2 poles (0.9844, -1.2348) (1.0067, -1.2373) (1.0192, -1.2373) knots 0 0 0 1 1 1
  spline S132 degree 2 poles (1.0192, -1.2373) (1.0962, -1.2373) (1.1833, -1.108) knots 0 0 0 1 1 1
  spline S133 degree 2 poles (1.1833, -1.108) (1.4592, -0.7102) (1.4592, -0.1732) knots 0 0 0 1 1 1
  spline S134 degree 2 poles (1.4592, -0.1732) (1.4592, 0.063) (1.402, 0.2445) knots 0 0 0 1 1 1
  spline S135 degree 2 poles (1.402, 0.2445) (1.3573, 0.3762) (1.1783, 0.5403) (1.0714, 0.5403) knots 0 0 0 1 2 2 2
  spline S136 degree 2 poles (1.0714, 0.5403) (0.8998, 0.5403) (0.8377, 0.3315) knots 0 0 0 1 1 1
  spline S137 degree 2 poles (0.8377, 0.3315) (0.8079, 0.2246) (0.7706, -0.1285) knots 0 0 0 1 1 1
  line L155 (0.7706, -0.1285) -> (0.7358, -0.479)
  spline S138 degree 2 poles (0.7358, -0.479) (0.701, -0.7898) (0.5866, -1.1776) (0.4797, -1.3268) knots 0 0 0 1 2 2 2
  spline S139 degree 2 poles (0.4797, -1.3268) (0.3703, -1.4784) (0.0148, -1.655) (-0.1891, -1.655) knots 0 0 0 1 2 2 2
  spline S140 degree 2 poles (-0.1891, -1.655) (-0.5098, -1.655) (-0.7609, -1.4461) knots 0 0 0 1 1 1
  spline S141 degree 2 poles (-0.7609, -1.4461) (-0.9896, -1.2597) (-1.099, -0.8644) knots 0 0 0 1 1 1
  spline S142 degree 2 poles (-1.099, -0.8644) (-1.1811, -0.5685) (-1.1811, -0.2329) knots 0 0 0 1 1 1
  spline S143 degree 2 poles (-1.1811, -0.2329) (-1.1811, 0.3737) (-0.8902, 0.9629) knots 0 0 0 1 1 1
  spline S144 degree 2 poles (-0.8902, 0.9629) (-0.833, 1.0873) (-0.833, 1.1121) knots 0 0 0 1 1 1
  spline S145 degree 2 poles (-0.833, 1.1121) (-0.833, 1.1419) (-0.8827, 1.2041) knots 0 0 0 1 1 1
  line L156 (-0.8827, 1.2041) -> (-0.8479, 1.2687)
  line L157 (-0.8479, 1.2687) -> (-0.1021, 0.9381)
  line L158 (-0.1021, 0.9381) -> (-0.1319, 0.8734)
  spline S146 degree 2 poles (-0.1319, 0.8734) (-0.1518, 0.8734) (-0.1617, 0.8734) knots 0 0 0 1 1 1
  spline S147 degree 2 poles (-0.1617, 0.8734) (-0.2612, 0.8734) (-0.3457, 0.7765) knots 0 0 0 1 1 1
  spline S148 degree 2 poles (-0.3457, 0.7765) (-0.4775, 0.6323) (-0.6639, 0.0257) (-0.6639, -0.2478) knots 0 0 0 1 2 2 2
  spline S149 degree 2 poles (-0.6639, -0.2478) (-0.6639, -0.5436) (-0.5645, -0.755) knots 0 0 0 1 1 1
  spline S150 degree 2 poles (-0.5645, -0.755) (-0.5073, -0.8693) (-0.3209, -1.0086) (-0.2214, -1.0086) knots 0 0 0 1 2 2 2
  spline S151 degree 2 poles (-0.2214, -1.0086) (-0.0698, -1.0086) (-0.0051, -0.8445) knots 0 0 0 1 1 1
  spline S152 degree 2 poles (-0.0051, -0.8445) (0.0396, -0.7326) (0.0794, -0.3845) knots 0 0 0 1 1 1
  line L159 (0.0794, -0.3845) -> (0.1142, -0.0415)
  spline S153 degree 2 poles (0.1142, -0.0415) (0.1515, 0.3041) (0.2162, 0.59) (0.2858, 0.7317) knots 0 0 0 1 2 2 2
  spline S154 degree 2 poles (0.2858, 0.7317) (0.3877, 0.9356) (0.5891, 1.0524) knots 0 0 0 1 1 1
  spline S155 degree 2 poles (0.5891, 1.0524) (0.7706, 1.1569) (1.0043, 1.1569) knots 0 0 0 1 1 1
  spline S156 degree 2 poles (1.0043, 1.1569) (1.3896, 1.1569) (1.6432, 0.8908) knots 0 0 0 1 1 1
  spline S157 degree 2 poles (1.6432, 0.8908) (1.9763, 0.5428) (1.9763, -0.1558) knots 0 0 0 1 1 1
  spline S158 degree 2 poles (1.9763, -0.1558) (1.9763, -0.4492) (1.857, -0.9539) (1.6979, -1.3293) knots 0 0 0 1 2 2 2
  spline S159 degree 2 poles (1.6979, -1.3293) (1.6482, -1.461) (1.6482, -1.4884) knots 0 0 0 1 1 1
  spline S160 degree 2 poles (1.6482, -1.4884) (1.6482, -1.5356) (1.6979, -1.5978) knots 0 0 0 1 1 1
  line L160 (1.6979, -1.5978) -> (1.6656, -1.6599)
  point P0 (-38.6989, -17.7144)
  constraints: 2 other
extrude "Extrusion6" cut sketch "Sketch9" against normal blind 25.4
body "Solid1"
